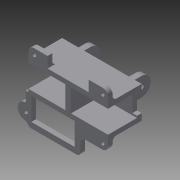
# Autodesk Inventor part: Motor_Enclosure
Saved by Autodesk Inventor 2015 (Build 190159000, 159)
## iProperties
Created: 2014-11-14
Part Number: Motor_Enclosure
Material: Generic
Document SubType Name: Modeling
Designer: s4201025
Density: 1 g/cm^3
Appearance: Default
Mass: 7.07047 g
Surface Area: 63.3593 cm^2
Volume: 7.07047 cm^3
Author: s4201025
Autodesk Inventor part; units mm, degrees
ref_plane "YZ Plane" through (0, 0, 0) normal (1, 0, 0) x (0, 1, 0)
ref_plane "XZ Plane" through (0, 0, 0) normal (0, 1, 0) x (-1, 0, 0)
sketch "Sketch1" plane through (0, 0, 0) normal (0, 1, 0) x (-1, 0, 0)
  circle A0 centre (-28.479, 37.72982) radius 1.0922
  circle A1 centre (-28.479, 19.62982) radius 1.0922
  line L0 (-32.729, 19.629821) -> (-32.729, 37.72982)
  arc A2 (-24.229, 37.72982) -> (-32.729, 37.72982) centre (-28.479, 37.72982) ccw
  arc A3 (-32.729, 19.533686) -> (-24.229, 19.533686) centre (-28.479, 19.533686) ccw
  line L1 (-21.229, 22.18177) -> (-21.229, 22.179821)
  line L2 (-21.229, 22.18177) -> (-21.229, 22.179821)
  line L3 (-21.229, 22.179821) -> (-21.229, 22.179821)
  line L4 (-24.229, 21.179821) -> (-21.229, 21.179821)
  line L5 (-24.229, 19.629821) -> (-24.229, 21.179821)
  line L6 (-21.229, 22.179821) -> (-21.229, 37.179821)
  circle A4 centre (-28.479, 19.62982) radius 1.0922
  arc A5 (-32.729, 19.629821) -> (-24.229, 19.629821) centre (-28.479, 19.629821) ccw
  line L7 (-24.229, 21.131769) -> (-21.229, 21.131769)
  line L8 (-21.229, 37.177872) -> (-21.229, 37.179821)
  line L9 (-21.229, 37.177872) -> (-21.229, 37.179821)
  circle A6 centre (-28.479, 37.72982) radius 1.0922
  arc A7 (-24.229, 37.72982) -> (-32.729, 37.72982) centre (-28.479, 37.72982) ccw
  line L10 (-21.229, 36.179821) -> (-24.229, 36.179821)
  line L11 (-24.229, 36.179821) -> (-21.229, 36.179821)
  line L12 (-32.729, 33.67982) -> (-32.729, 37.72982)
  line L13 (-24.229, 37.72982) -> (-24.229, 36.179821)
  line L14 (-24.229, 19.533686) -> (-24.229, 21.179821)
  line L15 (-24.229, 36.179821) -> (-24.229, 37.72982)
  line L16 (-8.729, 22.179821) -> (-21.229, 22.179821)
  line L17 (-21.229, 22.179821) -> (-21.229, 37.179821)
  line L18 (-1, 22.179821) -> (-8.729, 22.179821)
  circle A8 centre (28.479, 19.62982) radius 1.0922
  line L19 (21.229, 22.179821) -> (21.229, 39.97982)
  line L20 (21.229, 34.67982) -> (-21.229, 34.67982)
  line L21 (21.229, 24.67982) -> (-21.229, 24.67982)
  line L22 (8.729, 22.179821) -> (21.229, 22.179821)
  line L23 (21.229, 29.67982) -> (21.229, 22.147567)
  line L24 (21.229, 22.18177) -> (21.229, 22.147567)
  line L25 (21.229, 22.18177) -> (21.229, 22.147567)
  circle A9 centre (28.479, 37.72982) radius 1.0922
  line L26 (21.229, 37.177872) -> (21.229, 37.179821)
  line L27 (21.229, 34.67982) -> (21.229, 39.97982)
  line L28 (22.020904, 36.179821) -> (24.229, 36.179821)
  line L29 (24.229, 36.179821) -> (21.229, 36.179821)
  line L30 (24.229, 36.179821) -> (24.229, 37.72982)
  line L31 (24.229, 37.729821) -> (24.229, 36.179821)
  circle A10 centre (28.479, 37.72982) radius 1.0922
  arc A11 (32.729, 37.729821) -> (24.229, 37.72982) centre (28.479, 37.72982) ccw
  arc A12 (32.729, 37.729821) -> (24.229, 37.729821) centre (28.479, 37.729821) ccw
  line L32 (21.229, 37.177872) -> (21.229, 37.179821)
  arc A13 (24.229, 19.533686) -> (32.729, 19.533686) centre (28.479, 19.533686) ccw
  line L33 (24.229, 21.147567) -> (21.229, 21.147567)
  line L34 (24.229, 21.147567) -> (21.229, 21.147567)
  line L35 (24.229, 19.533686) -> (24.229, 21.147567)
  line L36 (24.229, 19.629821) -> (24.229, 21.147567)
  circle A14 centre (28.479, 19.62982) radius 1.0922
  arc A15 (24.229, 19.629821) -> (32.729, 19.629821) centre (28.479, 19.629821) ccw
  line L37 (32.729, 19.629821) -> (32.729, 37.729821)
  line L38 (-21.229, 22.179821) -> (21.229, 22.179821)
  line L39 (21.229, 22.18177) -> (21.229, 20.149516)
  line L40 (-21.229, 20.179821) -> (-21.229, 22.179821)
  line L41 (21.229, 20.179821) -> (21.229, 20.179821)
  line L42 (-21.229, 20.149516) -> (-21.229, 22.179821)
  line L43 (21.229, 20.179821) -> (21.229, 20.149516)
  line L44 (27.580166, 15.379821) -> (28.479, 15.379821)
  line L45 (-28.479, 15.379821) -> (-27.580166, 15.379821)
  line L46 (-18.229, 14.379821) -> (-3.5, 14.379821)
  arc A16 (-19.306033, 20.179821) -> (-18.229, 14.379821) centre (-18.229, 17.379821) ccw
  line L47 (-21.229, 39.17982) -> (-21.229, 39.97982)
  line L48 (21.229, 39.17982) -> (21.229, 39.97982)
  line L49 (-18.229, 42.97982) -> (18.229, 42.97982)
  arc A17 (-18.229, 42.97982) -> (-21.229, 39.97982) centre (-18.229, 39.97982) ccw
  arc A18 (21.229, 39.97982) -> (18.229, 42.97982) centre (18.229, 39.97982) ccw
  line L50 (21.229, 37.177872) -> (21.229, 39.97982)
  line L51 (-21.229, 39.97982) -> (-21.229, 34.67982)
  line L52 (-8.729, 37.177872) -> (-1.5, 37.177872)
  line L53 (17.157045, 37.177872) -> (21.229, 37.177872)
  line L54 (-21.229, 37.177872) -> (21.229, 37.177872)
  line L55 (21.229, 37.177872) -> (21.229, 34.67982)
  line L56 (21.229, 34.67982) -> (-21.229, 34.67982)
  line L57 (-21.229, 34.67982) -> (-21.229, 37.177872)
  line L58 (-21.229, 21.18177) -> (-21.229, 24.67982)
  line L59 (-21.229, 24.67982) -> (21.229, 24.67982)
  line L60 (21.229, 24.67982) -> (21.229, 22.18177)
  line L61 (-2, 37.177872) -> (-2, 37.179821)
  line L62 (-1.5, 37.177872) -> (-1.5, 37.179821)
  line L63 (1.5, 37.179821) -> (1.5, 37.177872)
  line L64 (2, 37.179821) -> (2, 37.177872)
  line L65 (-8.729, 37.177872) -> (-8.729, 37.179821)
  line L66 (-8.729, 37.179821) -> (-8.729, 37.177872)
  line L67 (8.729, 37.179821) -> (8.729, 37.177872)
  line L68 (8.729, 37.177872) -> (8.729, 37.179821)
  line L69 (-1.5, 24.67982) -> (-1.5, 34.67982)
  line L70 (1.5, 34.67982) -> (1.5, 24.67982)
  line L71 (-2, 34.67982) -> (2, 34.67982)
  line L72 (-2, 24.67982) -> (2, 24.67982)
  circle A19 centre (-18.229, 17.37982) radius 1.0922
  circle A20 centre (-18.229, 39.979819) radius 1.0922
  circle A21 centre (18.228999, 39.979819) radius 1.0922
  line L73 (-21.229, 24.67982) -> (-21.229, 22.67982)
  line L74 (-21.229, 22.67982) -> (21.229, 22.67982)
  line L75 (21.229, 22.67982) -> (21.229, 20.179821)
  line L76 (21.229, 20.179821) -> (-21.229, 20.179821)
  line L77 (-21.229, 20.179821) -> (-21.229, 22.67982)
  line L78 (21.229, 35.67982) -> (21.229, 38.17982)
  line L79 (-21.229, 38.17982) -> (-21.229, 35.67982)
  line L80 (-1.5, 37.177872) -> (1.5, 37.177872)
  line L81 (1.5, 34.67982) -> (1.5, 22.67982)
  line L82 (1.5, 22.67982) -> (-1.5, 22.67982)
  line L83 (-1.5, 22.67982) -> (-1.5, 34.67982)
  line L84 (-1.5, 28.67982) -> (5.646729, 28.67982)
  line L85 (-32.729, 28.67982) -> (32.729, 28.67982)
  line L86 (-21.229, 21.18177) -> (-3.5, 21.18177)
  line L87 (-21.229, 22.147567) -> (-3.5, 22.147567)
  line L88 (-3.5, 22.147567) -> (-3.5, 5.149516)
  line L89 (-3.5, 5.149516) -> (-21.229, 5.149516)
  line L90 (22.7, 21.147567) -> (22.7, 15.649516)
  line L91 (22.7, 21.147567) -> (21.229, 21.147567)
  line L92 (21.229, 21.147567) -> (21.229, 22.147567)
  line L93 (21.229, 5.149516) -> (-3.5, 5.149516)
  line L94 (19.7, 21.147567) -> (19.7, 7.149516)
  line L95 (22.7, 7.149516) -> (19.7, 7.149516)
  circle A22 centre (22.7, 11.399515) radius 1.0922
  circle A23 centre (22.7, 11.399515) radius 1.0922
  arc A24 (22.7, 7.149516) -> (22.7, 15.649516) centre (22.7, 11.399516) ccw
  arc A25 (22.7, 7.149516) -> (22.7, 15.649516) centre (22.7, 11.399516) ccw
  line L96 (22.7, 15.649516) -> (22.7, 21.147567)
  line L97 (-21.229, 20.149516) -> (21.229, 20.149516)
  line L98 (19.7, 20.149516) -> (-3.5, 20.149516)
  line L99 (-3.5, 20.179821) -> (-3.5, 5.149516)
  line L100 (-3.5, 8.149516) -> (19.7, 8.149516)
  line L101 (19.7, 8.149516) -> (19.7, 20.149516)
  line L102 (22.7, 21.147567) -> (19.7, 21.147567)
  line L103 (21.229, 22.67982) -> (-21.229, 22.67982)
  line L104 (21.229, 34.67982) -> (-21.229, 34.67982)
  line L105 (-21.229, 5.149516) -> (-21.229, 17.379821)
  line L106 (-21.229, 20.179821) -> (-21.229, 20.149516)
  line L107 (-21.229, 17.379821) -> (-21.229, 5.149516)
  line L108 (-21.229, 20.179821) -> (-21.229, 17.379821)
  line L109 (21.229, 5.149516) -> (21.229, 7.149516)
  line L110 (-3.5, 14.379821) -> (-6.5, 14.379821)
  line L111 (-6.5, 14.379821) -> (-6.5, 5.149516)
  line L112 (-6.5, 5.149516) -> (-3.5, 5.149516)
  line L113 (-3.5, 5.149516) -> (-3.5, 14.379821)
  line L114 (19.7, 20.179821) -> (21.229, 20.179821)
  line L115 (21.229, 20.179821) -> (21.229, 20.149516)
  line L116 (21.229, 20.149516) -> (19.7, 20.149516)
  line L117 (19.7, 20.149516) -> (19.7, 20.179821)
  line L118 (-11, 37.177872) -> (11, 37.177872)
  line L119 (11, 37.177872) -> (11, 111.177872)
  line L120 (11, 111.177872) -> (-11, 111.177872)
  line L121 (-11, 111.177872) -> (-11, 37.177872)
  line L122 (-13, 37.177872) -> (13, 37.177872)
  line L123 (13, 37.177872) -> (13, 113.177872)
  line L124 (13, 113.177872) -> (-13, 113.177872)
  line L125 (-13, 113.177872) -> (-13, 37.177872)
  line L126 (-13, 57.177872) -> (-11, 57.177872)
  line L127 (11, 57.177872) -> (13, 57.177872)
  line L128 (-11, 111.177872) -> (-11, 113.177872)
  line L129 (11, 111.177872) -> (11, 113.177872)
  point P0 (0, 0)
  point P1 (-19.04945, 20.533686)
  point P2 (-28.479, 41.979821)
  point P3 (8.729, 24.67982)
  point P4 (32.729, 33.67982)
  point P5 (32.729, 21.179821)
  point P6 (28.479, 41.979821)
  point P7 (-19.04945, 38.825954)
  point P8 (-19.04945, 38.825954)
  point P9 (19.04945, 38.825954)
  point P10 (19.04945, 38.825954)
  point P11 (21.229, 42.17982)
  point P12 (8.729, 34.67982)
  point P13 (2, 24.67982)
  point P14 (19.7, 20.149516)
  point P15 (-3.5, 20.149516)
  point P16 (26.95, 11.399516)
  point P17 (24.25289, 19.149516)
  point P18 (-24.229, 36.954821)
  point P19 (-24.229, 36.954821)
  point P20 (0, 28.67982)
  dimension "d5" = 15
  dimension "d40" = 42.458
  dimension "d112" = 2.5
  dimension "d139" = 12
  dimension "d157" = 12
  dimension "d158" = 23.2
  dimension "d163" = 12
  dimension "d185" = 22
  dimension "d186" = 74
  dimension "d187" = 26
  dimension "d188" = 76
  dimension "d190" = 20
  dimension "d207" = 11.5
  constraints: 258 end point, 50 point on line, 32 point on circle, 31 parallel, 26 centre point, 25 perpendicular, 13 horizontal, 7 midpoint, 2 tangent, 2 vertical, 15 other
  measures "d5" distance between parallel lines of L4 L10
  measures "d40" distance between parallel lines of L55 L57
  measures "d112" distance of L78.start L78.end
  measures "d139" distance between parallel lines of L74 L20
  measures "d157" distance between parallel lines of L100 L98
  measures "d158" distance between parallel lines of L99 L101
  measures "d163" distance between parallel lines of L103 L20
  measures "d185" distance of L120.end L119.end
  measures "d186" distance of L119.end L118.end
  measures "d187" distance of L124.end L123.end
  measures "d188" distance of L123.end L122.end
  measures "d207" distance between parallel lines of L0 L6
sketch "Sketch1 outline for Base_Extrusion" plane through (0, 0, 0) normal (0, 1, 0) x (-1, 0, 0)
  line L0 (-21.229, 20.179821) -> (-21.229, 17.379821)
  arc A0 (-18.229, 14.379821) -> (-21.229, 17.379821) centre (-18.229, 17.379821) cw
  line L1 (-6.5, 14.379821) -> (-18.229, 14.379821)
  line L2 (-6.5, 14.379821) -> (-6.5, 5.149516)
  line L3 (-6.5, 5.149516) -> (21.229, 5.149516)
  line L4 (21.229, 5.149516) -> (21.229, 7.149516)
  line L5 (21.229, 7.149516) -> (22.7, 7.149516)
  arc A1 (22.7, 7.149516) -> (22.7, 15.649516) centre (22.7, 11.399516) ccw
  line L6 (22.7, 15.649516) -> (22.7, 21.147567)
  line L7 (22.7, 21.147567) -> (21.229, 21.147567)
  line L8 (21.229, 20.179821) -> (21.229, 21.147567)
  line L9 (21.229, 20.179821) -> (19.7, 20.179821)
  line L10 (19.7, 20.179821) -> (19.7, 8.149516)
  line L11 (-3.5, 8.149516) -> (19.7, 8.149516)
  line L12 (-3.5, 8.149516) -> (-3.5, 20.149516)
  line L13 (-3.5, 20.149516) -> (-3.5, 20.179821)
  line L14 (-3.5, 20.179821) -> (-21.229, 20.179821)
  circle A2 centre (-18.229, 17.37982) radius 1.0922
  circle A3 centre (22.7, 11.399515) radius 1.0922
  line L15 (-21.229, 37.177872) -> (21.229, 37.177872)
  line L16 (21.229, 37.177872) -> (21.229, 39.97982)
  arc A4 (21.229, 39.97982) -> (18.229, 42.97982) centre (18.229, 39.97982) ccw
  line L17 (18.229, 42.97982) -> (-18.229, 42.97982)
  arc A5 (-18.229, 42.97982) -> (-21.229, 39.97982) centre (-18.229, 39.97982) ccw
  line L18 (-21.229, 39.97982) -> (-21.229, 37.177872)
extrude "Base_Extrusion" add sketch "Sketch1 outline for Base_Extrusion" along normal blind 2.5
sketch "Sketch1 outline for Side_Extrusion" plane through (0, 0, 0) normal (0, 1, 0) x (-1, 0, 0)
  line L0 (21.229, 22.67982) -> (1.5, 22.67982)
  line L1 (1.5, 22.67982) -> (1.5, 34.67982)
  line L2 (1.5, 34.67982) -> (21.229, 34.67982)
  line L3 (21.229, 34.67982) -> (21.229, 37.177872)
  line L4 (21.229, 37.177872) -> (-21.229, 37.177872)
  line L5 (-21.229, 37.177872) -> (-21.229, 34.67982)
  line L6 (-21.229, 34.67982) -> (-1.5, 34.67982)
  line L7 (-1.5, 34.67982) -> (-1.5, 22.67982)
  line L8 (-1.5, 22.67982) -> (-21.229, 22.67982)
  line L9 (-21.229, 22.67982) -> (-21.229, 20.179821)
  line L10 (-21.229, 20.179821) -> (21.229, 20.179821)
  line L11 (21.229, 20.179821) -> (21.229, 22.67982)
extrude "Side_Extrusion" add sketch "Sketch1 outline for Side_Extrusion" along normal blind 15.5
sketch "Sketch7" plane through (0, 15.5, 0) normal (0, 1, 0) x (1, 0, 0)
  line L0 (-21.229, -37.177872) -> (21.229, -37.177872)
  line L1 (21.229, -37.177872) -> (21.229, -22.177872)
  line L2 (21.229, -22.177872) -> (-21.229, -22.177872)
  line L3 (-21.229, -22.177872) -> (-21.229, -37.177872)
  point P0 (0, 0)
  dimension "d41" = 15
  constraints: 8 end point, 2 parallel, 1 horizontal, 1 perpendicular
  measures "d41" distance of L1.end L0.end
extrude "Extrusion11" add sketch "Sketch7" along normal blind 2.5
fillet "Fillet3" radius 2 3 edges at (0, 2.5, 37.1779) (12.3645, 2.5, 20.1798) (-20.4645, 2.5, 20.1798)
sketch "Sketch10" plane through (0, 18, 0) normal (0, 1, 0) x (1, 0, 0)
  line L0 (15, -34.67982) -> (-15, -34.67982)
  line L1 (-15, -24.67982) -> (15, -24.67982)
  line L2 (15, -34.67982) -> (-15, -34.67982)
  line L3 (-15, -34.67982) -> (-15, -24.67982)
  line L4 (-15, -24.67982) -> (15, -24.67982)
  line L5 (15, -34.67982) -> (15, -24.67982)
  line L6 (15, -34.67982) -> (12, -34.67982)
  line L7 (12, -34.67982) -> (12, -24.67982)
  line L8 (12, -24.67982) -> (15, -24.67982)
  line L9 (15, -24.67982) -> (15, -34.67982)
  line L10 (-15, -34.67982) -> (-12, -34.67982)
  line L11 (-12, -34.67982) -> (-12, -24.67982)
  line L12 (-12, -24.67982) -> (-15, -24.67982)
  line L13 (-15, -24.67982) -> (-15, -34.67982)
  point P0 (0, 0)
  dimension "d57" = 30
  dimension "d58" = 10
  dimension "d59" = 3
  dimension "d60" = 3
  constraints: 28 end point, 6 parallel, 4 horizontal, 4 perpendicular, 2 point on line
  measures "d57" distance of L1.start L4.end
  measures "d58" distance of L0.end L1.start
  measures "d59" distance of L7.end L8.end
  measures "d60" distance of L12.end L11.end
extrude "Extrusion15" add sketch "Sketch10" along normal blind 6 contours L0 L7 L1 L5 | L0 L3 L1 L11
sketch "Sketch11" plane through (15, 18, 34.67982) normal (1, 0, 0) x (0, 0, -1)
  line L0 (0, 6) -> (10, 6)
  line L1 (0, 0) -> (0, 6)
  arc A0 (10, 6) -> (0, 6) centre (5, 6) ccw
  circle A1 centre (5, 6) radius 1.5
  line L2 (-2.498052, -18) -> (0, -18)
  point P0 (34.67982, -18)
  dimension "d67" = 3
  dimension "d76" = 24
  dimension "d205" = 5
  constraints: 3 point on circle, 2 centre point, 1 coincident, 1 end point, 1 midpoint, 1 point on line
  measures "d67" diameter of A1
  measures "d76" distance from line of L2 L0.start
  measures "d205" distance of L0.end A0.centre
extrude "Extrusion16" add sketch "Sketch11" against normal blind 3 contours A1 L0 A0 | L0 A1 picked at (5.177302, 6.467508)
extrude "Extrusion17" cut sketch "Sketch11" against normal blind 3 contours A1 L0 | L0 A1
sketch "Sketch12" plane through (-15, 18, 24.67982) normal (-1, 0, 0) x (0, 0, 1)
  line L0 (0, 6) -> (10, 6)
  line L1 (0, 0) -> (0, 6)
  arc A0 (10, 6) -> (0, 6) centre (5, 6) ccw
  circle A1 centre (5, 6) radius 1.5
  line L2 (10, 0) -> (10, 6)
  line L3 (12.498052, -13.5) -> (12.498052, 0)
  line L4 (18.3, -18) -> (18.3, -15.5)
  line L5 (12.498052, 0) -> (-2.501948, 0)
  point P0 (-24.67982, -18)
  point P1 (34.67982, -14)
  dimension "d70" = 3
  dimension "d183" = 10
  dimension "d184" = 2.49805
  dimension "d206" = 13.3
  dimension "d209" = 6
  constraints: 5 end point, 3 point on circle, 2 centre point, 1 coincident, 1 midpoint, 1 point on line
  measures "d70" diameter of A1
  measures "d183" distance between parallel lines of L1 L2
  measures "d184" distance between parallel lines of L2 L3
  measures "d206" distance from line of L4 A0.centre
  measures "d209" distance from line of L5 A0.centre
extrude "Extrusion18" add sketch "Sketch12" against normal blind 3 contours A1 L0 A0 | L0 A1 picked at (5.177302, 6.467508)
extrude "Extrusion19" cut sketch "Sketch12" against normal blind 3 contours A1 L0 | L0 A1
fillet "Fillet4" radius 2 6 edges at (13.5, 18, 34.6798) (15, 18, 29.6798) (13.5, 18, 24.6798) (-13.5, 18, 34.6798) (-15, 18, 29.6798) (-13.5, 18, 24.6798)
sketch "Sketch17" plane through (0, 2.5, 0) normal (0, 1, 0) x (1, 0, 0)
  line L0 (-21.229, -5.179821) -> (6.5, -5.179821)
  line L1 (-19.7, -22.177872) -> (-22.7, -22.177872)
  line L2 (-22.7, -22.177872) -> (-19.7, -22.177872)
  line L3 (-19.7, -22.177872) -> (-19.7, -7.179821)
  line L4 (-22.7, -7.179821) -> (-19.7, -7.179821)
  circle A0 centre (-22.7, -11.42982) radius 1.0922
  circle A1 centre (-22.7, -11.42982) radius 1.0922
  arc A2 (-22.7, -7.179821) -> (-22.7, -15.679821) centre (-22.7, -11.429821) ccw
  arc A3 (-22.7, -7.179821) -> (-22.7, -15.679821) centre (-22.7, -11.429821) ccw
  line L5 (-22.7, -15.679821) -> (-22.7, -22.177872)
  line L6 (21.229, -20.179821) -> (-21.229, -20.179821)
  line L7 (-19.7, -20.179821) -> (3.5, -20.179821)
  line L8 (3.5, -20.179821) -> (3.5, -8.179821)
  line L9 (3.5, -8.179821) -> (-19.7, -8.179821)
  line L10 (-19.7, -8.179821) -> (-19.7, -20.179821)
  line L11 (-22.7, -21.177872) -> (-19.7, -21.177872)
  point P0 (0, 0)
  point P1 (-21.229, -22.177872)
  point P2 (-26.95, -11.429821)
  point P3 (0, -10.33762)
  point P4 (-24.25289, -20.179821)
  dimension "d132" = 5.1578
  dimension "d133" = 12
  dimension "d134" = 23.2
  constraints: 20 end point, 4 centre point, 4 parallel, 4 point on circle, 4 point on line, 2 perpendicular, 1 horizontal
  measures "d132" distance from line of point (0, -10.338) L0
  measures "d133" distance between parallel lines of L9 L7
  measures "d134" distance between parallel lines of L8 L10
sketch "Sketch18" plane through (0, 2.5, 0) normal (0, 1, 0) x (1, 0, 0)
  line L0 (21.229, -22.177872) -> (-21.229, -22.177872)
  line L1 (21.229, -22.177872) -> (3.5, -22.177872)
  line L2 (3.5, -22.177872) -> (3.5, -5.179821)
  line L3 (3.5, -5.179821) -> (21.229, -5.179821)
  line L4 (21.229, -5.179821) -> (21.229, -22.177872)
  line L5 (-22.7, -22.177872) -> (-22.7, -15.679821)
  line L6 (-22.7, -21.177872) -> (-21.229, -21.177872)
  line L7 (-21.229, -21.177872) -> (-21.229, -22.177872)
  line L8 (-21.229, -22.177872) -> (-22.7, -22.177872)
  line L9 (-22.7, -22.177872) -> (-22.7, -21.177872)
  point P0 (-19.7, -20.179821)
  point P1 (3.5, -20.179821)
  point P2 (21.229, -19.379821)
  point P3 (11.5, -13.129821)
  point P4 (-22.7, -22.147567)
  constraints: 16 end point, 4 parallel, 2 horizontal, 2 perpendicular, 1 point on line
extrude "Extrusion28" add sketch "Sketch1" along normal blind 18 contours L74 L19 L22 L38 L18 L16 L6 | L16 L18 L38 L22 L23 L39 L102 L94 L76 L88 L87 L40 | L87 L88 L86 L40 | L40 L86 L88 L76 | L94 L102 L39 L76
extrude "Extrusion30" [suppressed]
extrude "Extrusion31" cut sketch "Sketch17" against normal blind 10 and the other way blind 5 contours L3 L9 L8 L6
extrude "Extrusion26" cut sketch "Sketch1" along normal mid plane 10 contours A19 | A20 | A21 | A22
extrude "Extrusion33" cut sketch "Sketch18" against normal blind 3 contours L5 L6 L7 L8
fillet "Fillet10" radius 2 4 edges at (6.5, 1.25, 14.3798) (6.5, 1.25, 5.1495) (-21.229, 1.25, 5.1495) (-21.229, 1.25, 7.1495)
sketch "Sketch24" plane through (-21.229, 0, 39.97982) normal (-1, 0, 0) x (0, 0, 1)
  line L0 (-16.3, 18) -> (-6.3, 18)
  line L1 (-6.3, 18) -> (-6.3, 15.5)
  line L2 (-6.3, 15.5) -> (-16.3, 15.5)
  line L3 (-16.3, 15.5) -> (-16.3, 18)
  point P0 (-39.97982, 0)
  dimension "d169" = 10
  constraints: 8 end point, 2 parallel, 1 horizontal, 1 perpendicular
  measures "d169" distance of L1.end L2.end
extrude "Extrusion35" cut sketch "Sketch24" against normal blind 2.5
sketch "Sketch25" plane through (21.229, 0, 39.97982) normal (1, 0, 0) x (0, 0, -1)
  line L0 (6.3, 15.5) -> (16.3, 15.5)
  line L1 (16.3, 15.5) -> (16.3, 18)
  line L2 (16.3, 18) -> (6.3, 18)
  line L3 (6.3, 18) -> (6.3, 15.5)
  line L4 (17.3, 0) -> (17.3, 15.5) projected
  line L5 (5.3, 0) -> (5.3, 15.5) projected
  line L6 (5.3, 0) -> (17.3, 0) projected
  point P0 (39.97982, 0)
  point P1 (17.3, 2.5)
  point P2 (15.3, 0)
  dimension "d173" = 10
  dimension "d174" = 12
  dimension "d175" = 15.5
  constraints: 8 end point, 2 parallel, 1 horizontal, 1 perpendicular
  measures "d173" distance of L2.end L1.end
  measures "d174" distance between parallel lines of L4 L5
  measures "d175" distance between parallel lines of L0 L6
extrude "Extrusion36" cut sketch "Sketch25" against normal blind 2.5
sketch "Sketch26" plane through (0, 18, 0) normal (0, 1, 0) x (1, 0, 0)
  line L0 (15, -24.67982) -> (15, -34.67982)
  line L1 (18.729, -23.67982) -> (18.729, -33.67982)
  line L2 (12, -36.67982) -> (12, -22.67982)
  line L3 (12, -29.67982) -> (18.729, -29.67982)
  line L4 (18.729, -33.67982) -> (18.729, -23.67982)
  point P0 (0, 0)
  point P1 (15, -29.67982)
  point P2 (18.729, -28.67982)
  dimension "d178" = 1
  constraints: 3 midpoint, 2 end point, 1 perpendicular, 1 point on line
  measures "d178" distance of L3.end point (18.729, -28.68)
sketch "Sketch27" plane through (0, 18, 0) normal (0, 1, 0) x (1, 0, 0)
  line L0 (12, -24.67982) -> (12, -34.67982)
  line L1 (21.229, -37.177872) -> (21.229, -33.67982)
  line L2 (15, -24.67982) -> (15, -34.67982)
  point P0 (0, 0)
  dimension "d182" = 3
  measures "d182" distance between parallel lines of L0 L2
extrude "Extrusion37" cut sketch "Sketch1" along normal blind 10 contours L121 L49 L119 L54 L52 | L121 L120 L119 L49
ref_plane "Work Plane3" through (-15, 29, 29.67982) normal (0, -1, 0) x (1, 0, 0)
sketch "Sketch29" plane through (-15, 29, 29.67982) normal (0, -1, 0) x (1, 0, 0)
  line L0 (36.229, -6) -> (36.229, -9.5) projected
  line L1 (-6.229, -9.5) -> (-6.229, -6) projected
  point P0 (15, -29.67982)
  dimension "d208" = 42.458
  measures "d208" distance between parallel lines of L0 L1
body "Solid2"
